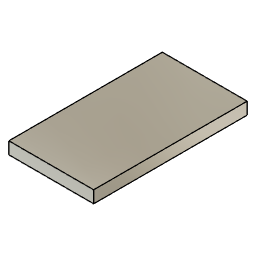
OpenBook_device_fusion (Autodesk Fusion 360 archive; units mm, degrees)
design "Battery"
Autodesk Fusion 360 part; units mm, degrees
sketch "Sketch1" plane through (0, 0, 0) normal (0, 0, 1) x (1, 0, 0)
  line L0 (0, 0) -> (42, 0)
  line L1 (42, 0) -> (42, 76)
  line L2 (42, 76) -> (0, 76)
  line L3 (0, 76) -> (0, 0)
  dimension "d3" = 42
  dimension "d4" = 76
  constraint horizontal L0
  constraint vertical L1
  constraint horizontal L2
  constraint vertical L3
  constraint coincident L0.start L3.end
  measures "d3" distance of L0.start L0.end
  measures "d4" distance of L0.start L2.end
extrude "Extrude1" add sketch "Sketch1" along normal blind 6

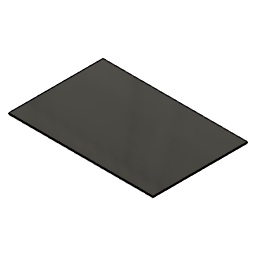
design "Display"
Autodesk Fusion 360 part; units mm, degrees
sketch "Sketch1" plane through (0, 0, 0) normal (0, 0, 1) x (1, 0, 0)
  line L0 (0, 0) -> (170.2, 0)
  line L1 (170.2, 0) -> (170.2, 111.2)
  line L2 (170.2, 111.2) -> (0, 111.2)
  line L3 (0, 111.2) -> (0, 0)
  dimension "d1" = 170.2
  dimension "d2" = 111.2
  constraint horizontal L0
  constraint vertical L1
  constraint horizontal L2
  constraint vertical L3
  constraint coincident L0.start L3.end
  measures "d1" distance of L0.start L0.end
  measures "d2" distance of L0.start L2.end
extrude "Extrude1" add sketch "Sketch1" along normal blind 1.18
